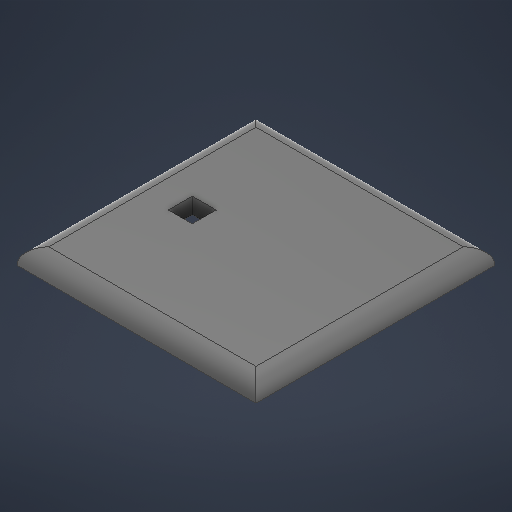
# Autodesk Inventor part: podstawa
Saved by Autodesk Inventor 2027 (Build 310192060, 192F)
## iProperties
Created: 2026-08-24
Part Number: podstawa
Material: Ogólny
Document SubType Name: Modeling
Designer: User
Density: 1 g/cm^3
Appearance: Domyślna
Author: User
Autodesk Inventor part; units mm, degrees
ref_plane "YZ Plane" through (0, 0, 0) normal (1, 0, 0) x (0, 1, 0)
ref_plane "XZ Plane" through (0, 0, 0) normal (0, 1, 0) x (-1, 0, 0)
ref_plane "XY Plane" through (0, 0, 0) normal (0, 0, 1) x (1, 0, 0)
sketch "Szkic1" plane through (0, 0, 0) normal (0, 1, 0) x (-1, 0, 0)
  line L0 (-75, 75) -> (75, 75)
  line L1 (75, 75) -> (75, -75)
  line L2 (75, -75) -> (-75, -75)
  line L3 (-75, -75) -> (-75, 75)
  line L4 (-75, 75) -> (75, -75) construction
  line L5 (75, 75) -> (-75, -75) construction
  line L6 (-10, 10) -> (10, -10) construction
  line L7 (10, 10) -> (-10, -10) construction
  line L8 (0, 0) -> (40, 0)
  line L9 (0, 0) -> (40, 0) construction
  line L10 (47.5, 7.5) -> (32.5, 7.5)
  line L11 (32.5, 7.5) -> (32.5, -7.5)
  line L12 (32.5, -7.5) -> (47.5, -7.5)
  line L13 (47.5, -7.5) -> (47.5, 7.5)
  line L14 (47.5, 7.5) -> (32.5, -7.5) construction
  line L15 (32.5, 7.5) -> (47.5, -7.5) construction
  dimension "d0" = 150
  dimension "d1" = 150
  dimension "d7" = 40
  dimension "d8" = 0
  dimension "d9" = 15
  dimension "d10" = 15
  constraints: 32 end point, 6 midpoint, 4 horizontal, 4 parallel, 2 perpendicular, 1 collinear
  measures "d0" distance of L1.end L2.end
  measures "d1" distance of L0.end L1.end
  measures "d7" distance of L8.start L8.end
  measures "d8" distance between parallel lines of L8 L9
  measures "d9" distance of L12.end L11.end
  measures "d10" distance of L11.end L10.end
extrude "Wyciągnięcie proste1" add sketch "Szkic1" along normal blind 10
fillet "Zaokrąglenie1" radius 10 4 edges at (0, 10, 75) (75, 10, 0) (0, 10, -75) (-75, 10, 0)
